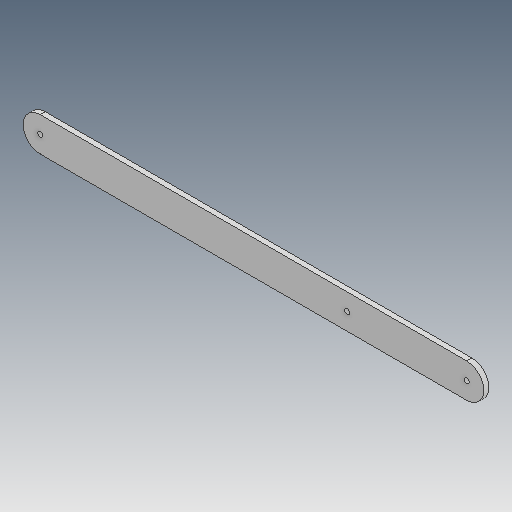
# Autodesk Inventor part: Träger vorne oben lang
Saved by Autodesk Inventor 2020 (Build 240168000, 168)
## iProperties
Created: 2021-06-29
Part Number: Träger vorne oben lang
Material: Generisch
Document SubType Name: Modeling
Designer: Mike
Density: 1 g/cm^3
Appearance: Vorgabe
Author: Mike
Autodesk Inventor part; units mm, degrees
ref_plane "YZ Plane" through (0, 0, 0) normal (1, 0, 0) x (0, 1, 0)
ref_plane "XZ Plane" through (0, 0, 0) normal (0, 1, 0) x (-1, 0, 0)
ref_plane "XY Plane" through (0, 0, 0) normal (0, 0, 1) x (1, 0, 0)
sketch "Skizze1" plane through (0, 0, 0) normal (0, 0, 1) x (1, 0, 0)
  line L0 (-189.879, 0) -> (188.121, 0) projected
  line L1 (0, -8.5091) -> (0, 51.0549) projected
  line L2 (-125.879, 42.5457) -> (124.121, 42.5457)
  line L3 (124.121, 22.5457) -> (-125.879, 22.5457)
  arc A0 (-125.879, 42.5457) -> (-125.879, 22.5457) centre (-125.879, 32.5457) ccw
  arc A1 (124.121, 22.5457) -> (124.121, 42.5457) centre (124.121, 32.5457) ccw
  point P0 (0, 0)
  dimension "d5" = 250
  dimension "d6" = 20
  constraints: 4 end point, 4 point on circle, 4 point on line, 2 centre point, 1 horizontal, 1 parallel
  measures "d5" distance of L2.start L2.end
  measures "d6" distance between parallel lines of L2 L3
extrude "Extrusion1" add sketch "Skizze1" along normal blind 3
sketch "Skizze2" plane through (0, 0, 3) normal (0, 0, 1) x (1, 0, 0)
  arc A0 (124.121, 22.5457) -> (124.121, 42.5457) centre (124.121, 32.5457) ccw projected
  line L0 (124.121, 42.5457) -> (-125.879, 42.5457) projected
  arc A1 (-125.879, 42.5457) -> (-125.879, 22.5457) centre (-125.879, 32.5457) ccw projected
  point P0 (0, 0)
  point P1 (-125.879, 32.5457)
  dimension "d9" = 10
  dimension "d10" = 0
  constraints: 1 coincident
  measures "d9" distance from line of L0 point (-125.879, 32.546)
  measures "d10" distance of A1.centre point (-125.879, 32.546)
hole "Bohrung1" at (-125.879, 32.5457, 3) at (124.121, 32.5457, 3) direction (0, 0, -1) diameter 3 depth 57.1 tip angle 118
sketch "Skizze3" plane through (0, 0, 3) normal (0, 0, 1) x (1, 0, 0)
  circle A0 centre (124.121, 32.5457) radius 1.5 projected
  line L0 (124.121, 42.5457) -> (-125.879, 42.5457) projected
  point P0 (0, 0)
  point P1 (54.121, 32.5457)
  dimension "d18" = 70
  dimension "d19" = 10
  measures "d18" distance of A0.centre point (54.121, 32.546)
  measures "d19" distance from line of L0 point (54.121, 32.546)
hole "Bohrung2" at (54.121, 32.5457, 3) direction (0, 0, -1) diameter 3 depth 57.1 tip angle 118
